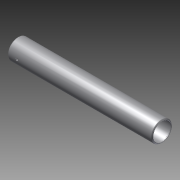
# Autodesk Inventor part: 04-5.6362C
Saved by Autodesk Inventor 2012 (Build 160160000, 160)
## iProperties
Created: 2013-01-17
Part Number: 04-5.6362C
Material: Default
Catalog Web Link: www.cadenas.de
Description: Tube-Original Line - Standard Air Cylinders
Vendor: BIMBA
Document SubType Name: Modeling
Designer: William
Manufacturer: BIMBA
Density: 1 g/cm^3
Category: PARTsolutions
Company: BIMBA
Title: 04-5.6362C
Author: Cadenas PARTsolutions
Comments: Original Line - Standard Air Cylinders
PSOL_IDENT_0: {\\10.0.0.242\data_v9\23d-libs\bimba\bimba\bimba_imperial\bimba_full_line\original_line_cylinders\st
PSOL_IDENT_1: andard_air_cylinders\tube.prj},188 {VTYP=3D},{NB=04-5.6362C},{LINA=04-5.6362C},{NN=Tube},{DATE=20.08
PSOL_IDENT_2: .2011 07:16:50},{GEOMDATE=18.02.2011 00:00:00},{VERSION=},{LINEID=40},{LINESUBID=-1},{WBVAR=MNT,ACTI
PSOL_IDENT_3: NG,NR,L,FOURHOLES,SR}  {NB=04-5.6362C},{LINA=04-5.6362C},{KT=DUMMY},{PN=04-5.6362C},{BORE=0.75000000
PSOL_IDENT_4: },{BOREPN=04},{MNT=},{MNTALG='' , 'Front Nose' , 'BF' , 'Front Block' , 'BFT' , 'Front Trunnion' , '
PSOL_IDENT_5: A' , 'Adjustable Stroke'},{ACTING=},{ACTINGALG= '' , 'Single Acting' , 'R' , 'Reverse/Double Acting'
PSOL_IDENT_6: },{NR=},{NRALG= '' , 'Without Non-rotating Rod' , 'NR' , 'With Non-rotating Rod' },{L=5.6360},{OD=0
PSOL_IDENT_7: .8050},{ODN=0.8050},{ODP=0.8625},{ODB=0.8325},{ID=0.7615},{DV=0.00000000},{LV=0.00000000},{LV1=0.000
PSOL_IDENT_8: 00000},{G=0.0300},{FOURHOLES=2},{AA=0.3750},{BB=0.0940},{SR=C},{SRALG= 'C' , 'Carbon Steel Rod' , 'S
PSOL_IDENT_9: R' , '303 Stainless Steel Rod' , '' , '303 Stainless Steel Rod'}
CNS_NT: Original Line - Standard Air Cylinders
CNS_NB: 04-5.6362C
CNS_NBSYN: $PN.
CNS_LINA: 04-5.6362C
CNS_PN: 04-5.6362C
CNS_BORE: 3/4
CNS_BOREPN: 04
CNS_MNT: Front Nose
CNS_MNTALG: '' , 'Front Nose' , 'BF' , 'Front Block' , 'BFT' , 'Front Trunnion' , 'A' , 'Adjustable Stroke'
CNS_ACTING: Single Acting
CNS_ACTINGALG: '' , 'Single Acting' , 'R' , 'Reverse/Double Acting'
CNS_NR: Without Non-rotating Rod
CNS_NRALG: '' , 'Without Non-rotating Rod' , 'NR' , 'With Non-rotating Rod'
CNS_L: 5.6360
CNS_OD: 0.8050
CNS_ODN: 0.8050
CNS_ODP: 0.8625
CNS_ODB: 0.8325
CNS_ID: 0.7615
CNS_DV: 0.00000000
CNS_LV: 0.00000000
CNS_LV1: 0.00000000
CNS_G: 0.0300
CNS_FOURHOLES: 2
CNS_AA: 0.3750
CNS_BB: 0.0940
CNS_SR: Carbon Steel Rod
CNS_SRALG: 'C' , 'Carbon Steel Rod' , 'SR' , '303 Stainless Steel Rod' , '' , '303 Stainless Steel Rod'
SUPPLIER: BIMBA
ARTICLENO: 04-5.6362C
BOMINFO: 04-5.6362C
CREATOR: CADENAS GmbH
Autodesk Inventor part; units mm, degrees
sketch "Sketch_1" plane through (0, 0, 0) normal (0, 0, 1) x (1, 0, 0)
  line L0 (143.1544, 0) -> (0, 0)
  arc A0 (-0.6395, 9.3472) -> (-0.6395, 9.1676) centre (-0.5497, 9.2574) ccw
  line L1 (-0.6395, 9.1676) -> (-0.381, 8.9091)
  line L2 (-0.381, 8.9091) -> (0, 8.9091)
  line L3 (0, 8.9091) -> (0.762, 9.671)
  line L4 (0.762, 9.671) -> (142.3924, 9.671)
  line L5 (142.3924, 9.671) -> (143.1544, 8.9091)
  line L6 (143.1544, 8.9091) -> (143.5354, 8.9091)
  line L7 (143.5354, 8.9091) -> (143.7939, 9.1676)
  arc A1 (143.7939, 9.1676) -> (143.7939, 9.3472) centre (143.7041, 9.2574) ccw
  line L8 (143.7939, 9.3472) -> (143.1408, 10.0003)
  arc A2 (143.1408, 10.0003) -> (142.6019, 10.2235) centre (142.602, 9.4615) ccw
  line L9 (142.6019, 10.2235) -> (0.5524, 10.2235)
  arc A3 (0.5524, 10.2235) -> (0.0136, 10.0003) centre (0.5524, 9.4615) ccw
  line L10 (0.0136, 10.0003) -> (-0.6395, 9.3472)
  constraints: 22 end point, 8 point on circle, 4 centre point
revolve "Revolution1" add sketch "Sketch_1" angle 360 about axis through (143.1544, 0, 0) along (1, 0, 0)
sketch "Sketch_4" plane through (0, 0, 0) normal (0, 0, 1) x (1, 0, 0)
  circle A0 centre (8.763, 0) radius 1.1938
  constraints: 1 centre point
extrude "Extrusion1" cut sketch "Sketch_4" along normal blind 10.2235
ref_plane "tube_front_XY" through (0, 0, 0) normal (1, 0, 0) x (0, 0, -1)
ref_plane "tube_front_YZ" through (0, 0, 0) normal (0, 0, -1) x (0, 1, 0)
ref_plane "tube_front_ZX" through (0, 0, 0) normal (0, 1, 0) x (1, 0, 0)
ref_plane "tube_rear_XY" through (143.1544, 0, 0) normal (1, 0, 0) x (0, 0, -1)
ref_plane "tube_rear_YZ" through (143.1544, 0, 0) normal (0, 0, -1) x (0, 1, 0)
ref_plane "tube_rear_ZX" through (143.1544, 0, 0) normal (0, 1, 0) x (1, 0, 0)
ref_plane "cp1_XY" through (71.5772, 10.2235, 0) normal (1, 0, 0) x (0, 0, -1)
ref_plane "cp1_YZ" through (71.5772, 10.2235, 0) normal (0, 0, -1) x (0, 1, 0)
ref_plane "cp1_ZX" through (71.5772, 10.2235, 0) normal (0, 1, 0) x (1, 0, 0)
ref_plane "cp2_XY" through (71.5772, 0, -10.2235) normal (1, 0, 0) x (0, 0, -1)
ref_plane "cp2_YZ" through (71.5772, 0, -10.2235) normal (0, 0, -1) x (0, 1, 0)
ref_plane "cp2_ZX" through (71.5772, 0, -10.2235) normal (0, 1, 0) x (1, 0, 0)
ref_plane "cp3_XY" through (71.5772, -10.2235, 0) normal (1, 0, 0) x (0, 0, -1)
ref_plane "cp3_YZ" through (71.5772, -10.2235, 0) normal (0, 0, -1) x (0, 1, 0)
ref_plane "cp3_ZX" through (71.5772, -10.2235, 0) normal (0, 1, 0) x (1, 0, 0)
ref_plane "cp4_XY" through (71.5772, 0, 10.2235) normal (1, 0, 0) x (0, 0, -1)
ref_plane "cp4_YZ" through (71.5772, 0, 10.2235) normal (0, 0, -1) x (0, 1, 0)
ref_plane "cp4_ZX" through (71.5772, 0, 10.2235) normal (0, 1, 0) x (1, 0, 0)
body "Solid1"
